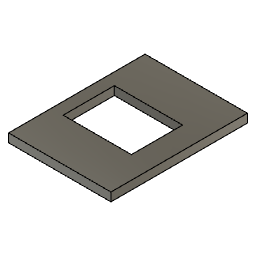
Perfboard Power System Floor (Autodesk Fusion 360 design; units mm, degrees)
Autodesk Fusion 360 part; units mm, degrees
sketch "Sketch1" plane through (0, 0, 0) normal (0, 0, 1) x (1, 0, 0)
  line L0 (0, 0) -> (60, 0)
  line L1 (60, 0) -> (60, -80)
  line L2 (60, -80) -> (0, -80)
  line L3 (0, -80) -> (0, 0)
  line L4 (7, -25) -> (47, -25)
  line L5 (47, -25) -> (47, -55)
  line L6 (47, -55) -> (7, -55)
  line L7 (7, -55) -> (7, -25)
  dimension "d7" = 60
  dimension "d8" = 80
  dimension "d15" = 40
  dimension "d16" = 30
  dimension "d17" = 7
  dimension "d18" = 25
  constraint horizontal L0
  constraint vertical L1
  constraint horizontal L2
  constraint vertical L3
  constraint coincident L0.start L3.end
  constraint horizontal L4
  constraint vertical L5
  constraint horizontal L6
  constraint vertical L7
  measures "d7" distance of L0.start L0.end
  measures "d8" distance of L0.start L2.end
  measures "d15" distance of L4.start L4.end
  measures "d16" distance of L4.start L6.end
  measures "d17" distance of L3 L7
  measures "d18" distance of L0 L4
extrude "Extrude1" add sketch "Sketch1" along normal blind 5 contours L0 L1 L2 L3 | L4 L5 L6 L7
extrude "Extrude2" cut sketch "Sketch1" along normal blind 100 contours L4 L5 L6 L7
equation "perfboard_length = 60 mm"
equation "perfboard_width = 40 mm"
equation "width = perfboard_length + 2 * screw_radius * 2"
equation "length = perfboard_width + 2 * screw_radius * 2"
equation "height = 5 mm"
equation "d7 = length"
equation "d8 = width"
equation "d9 = height"
equation "middle_gap_width = 30 mm"
equation "middle_gap_length = length - 2 * screw_radius * 2"
equation "middle_gap_small_distance = 7 mm"
equation "middle_gap_big_distance = ( width - middle_gap_width ) / 2"
equation "d15 = middle_gap_length"
equation "d16 = middle_gap_width"
equation "d17 = middle_gap_small_distance"
equation "d18 = middle_gap_big_distance"
equation "extra = 100 mm"
equation "d20 = extra"
equation "screw_radius = 5 mm"
